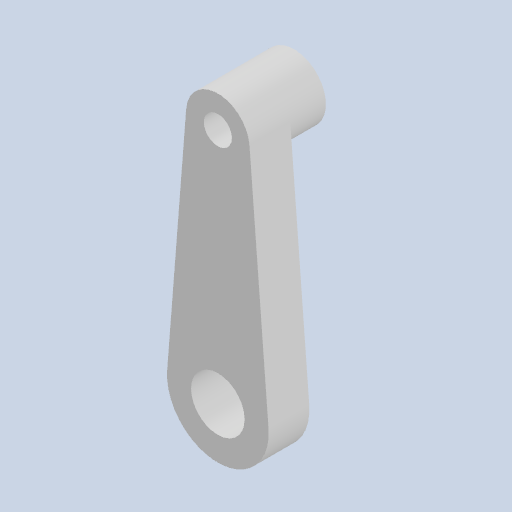
# Autodesk Inventor part: shatun
Saved by Autodesk Inventor 2022 (Build 260153000, 153)
## iProperties
Created: 2024-10-19
Part Number: shatun
Material: Типовые
Document SubType Name: Modeling
Designer: Andrey
Density: 1 g/cm^3
Appearance: По умолчанию
Author: Andrey
Autodesk Inventor part; units mm, degrees
ref_plane "YZ Plane" through (0, 0, 0) normal (1, 0, 0) x (0, 1, 0)
ref_plane "XZ Plane" through (0, 0, 0) normal (0, 1, 0) x (-1, 0, 0)
ref_plane "XY Plane" through (0, 0, 0) normal (0, 0, 1) x (1, 0, 0)
sketch "Эскиз1" plane through (0, 0, 0) normal (0, 0, 1) x (1, 0, 0)
  circle A0 centre (0, 10.0167) radius 1.6 projected
  line L0 (25.2327, 9.549) -> (31.7335, -1.7106) projected
  arc A1 (11.3933, 4.2802) -> (25.2327, 9.549) centre (0, 55.0167) ccw projected
  line L1 (11.3933, 4.2802) -> (2.8284, 12.8451) projected
  arc A2 (2.8284, 12.8451) -> (-2.8284, 12.8451) centre (0, 10.0167) ccw projected
  line L2 (-2.8284, 12.8451) -> (-11.3933, 4.2802) projected
  arc A3 (-25.2327, 9.549) -> (-11.3933, 4.2802) centre (0, 55.0167) ccw projected
  line L3 (-31.7335, -1.7106) -> (-25.2327, 9.549) projected
  arc A4 (-31.7335, -1.7106) -> (31.7335, -1.7106) centre (0, 55.0167) ccw projected
  arc A5 (1.9935, 28.8226) -> (-1.9935, 28.8226) centre (0, 28.6617) ccw projected
  line L4 (-1.9935, 28.8226) -> (-3.4887, 10.2982) projected
  arc A6 (-3.4887, 10.2982) -> (3.4887, 10.2982) centre (0, 10.0167) ccw projected
  line L5 (3.4887, 10.2982) -> (1.9935, 28.8226) projected
  circle A7 centre (0, 28.6617) radius 1.1 projected
  circle A8 centre (0, 10.0167) radius 0.95 projected
  circle A9 centre (0, 28.6617) radius 1.6
  circle A10 centre (0, 10.0167) radius 2.1
  circle A11 centre (0, 10.0167) radius 4
  circle A12 centre (0, 28.6617) radius 2.5
  line L6 (-2.4919, 28.8628) -> (-3.987, 10.3385)
  line L7 (3.987, 10.3385) -> (2.4919, 28.8628)
  point P0 (0, 0)
  dimension "d0" = 3.2
  dimension "d1" = 4.2
  dimension "d2" = 8
  dimension "d3" = 5
  constraints: 4 centre point, 4 coincident, 4 end point, 4 point on circle, 4 tangent
  measures "d0" diameter of A9
  measures "d1" diameter of A10
  measures "d2" diameter of A11
  measures "d3" diameter of A12
extrude "Выдавливание1" add sketch "Эскиз1" along normal blind 3.2 contours L7 A11 L5 L1 | L1 L5 A12 L7 | L5 A11 L1 | L1 A2 L2 L4 A12 L5 | A11 L4 A6 L5 | A12 L5 A5 L4 | A11 L5 A6 L4 A2 | A12 L4 A5 L5 | A12 L4 L2 L6 | L2 L4 A11 L6 | A11 L4 L2 | A9
sketch "Эскиз2" plane through (0, 0, 0) normal (0, 0, -1) x (-1, 0, 0)
  line L0 (0, 6.9767) -> (0, 71.9606) projected
  line L1 (-1.9935, 28.8226) -> (-3.4887, 10.2982) projected
  arc A0 (-3.4887, 10.2982) -> (3.4887, 10.2982) centre (0, 10.0167) ccw projected
  line L2 (3.4887, 10.2982) -> (1.9935, 28.8226) projected
  arc A1 (1.9935, 28.8226) -> (-1.9935, 28.8226) centre (0, 28.6617) ccw projected
  circle A2 centre (0, 10.0167) radius 1.925 projected
  circle A3 centre (0, 28.6617) radius 1.1 projected
  circle A4 centre (0, 28.6617) radius 1.1 projected
  circle A5 centre (0, 10.0167) radius 2.1 projected
  arc A6 (-3.987, 10.3385) -> (3.987, 10.3385) centre (0, 10.0167) ccw projected
  line L3 (2.4919, 28.8628) -> (3.987, 10.3385) projected
  arc A7 (2.4919, 28.8628) -> (-2.4919, 28.8628) centre (0, 28.6617) ccw projected
  line L4 (-3.987, 10.3385) -> (-2.4919, 28.8628) projected
  circle A8 centre (0, 28.6617) radius 2.5
  point P0 (0, 0)
  point P1 (-2.4919, 28.8628)
  constraints: 1 centre point, 1 coincident, 1 tangent
extrude "Выдавливание2" add sketch "Эскиз2" along normal blind 2.8 contours A8 L1 A1 L0 A3 | L0 A3 A1 L2 A8 | A8 A7 L0 A1 L1 | L2 A1 L0 A7 A8
